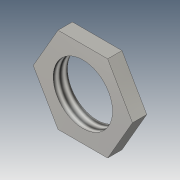
# Autodesk Inventor part: Porca do Plug P10
Saved by Autodesk Inventor 2016 (Build 200138000, 138)
## iProperties
Created: 2018-12-01
Part Number: Porca do Plug P10
Material: Generic
Document SubType Name: Modeling
Designer: Pedro Mendonça
Density: 1 g/cm^3
Appearance: Aluminum - Polished
Author: Pedro Mendonça
Autodesk Inventor part; units mm, degrees
ref_plane "YZ Plane" through (0, 0, 0) normal (1, 0, 0) x (0, 1, 0)
ref_plane "XZ Plane" through (0, 0, 0) normal (0, 1, 0) x (-1, 0, 0)
ref_plane "XY Plane" through (0, 0, 0) normal (0, 0, 1) x (1, 0, 0)
sketch "Sketch1" plane through (0, 0, 0) normal (1, 0, 0) x (0, 1, 0)
  line L0 (6.9282, 0) -> (3.4641, -6)
  line L1 (3.4641, -6) -> (-3.4641, -6)
  line L2 (-3.4641, -6) -> (-6.9282, 0)
  line L3 (-6.9282, 0) -> (-3.4641, 6)
  line L4 (-3.4641, 6) -> (3.4641, 6)
  line L5 (3.4641, 6) -> (6.9282, 0)
  circle A0 centre (0, 0) radius 4.15
  dimension "d0" = 12
  dimension "d1" = 8.3
  constraints: 12 end point, 2 coincident, 1 centre point, 13 other
  measures "d0" distance between parallel lines of L1 L4
  measures "d1" diameter of A0
extrude "Extrusion1" add sketch "Sketch1" along normal mid plane 2
thread "Thread1" size "M8x1" class "6H" standard "ANSI Metric M Profile" full length
body "Solid1"
